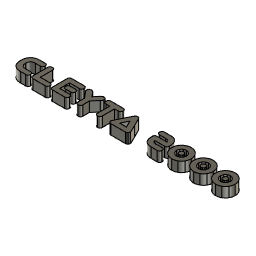
cleyta - letras v1 (Autodesk Fusion 360 design; units mm, degrees)
Autodesk Fusion 360 part; units mm, degrees
sketch "Sketch1" plane through (0, 0, 0) normal (0, 0, 1) x (1, 0, 0)
  spline S0 degree 3 poles (59.1791, -37.5966) (59.1791, -37.7184) (59.1478, -37.8357) (59.086, -37.9476) knots 0 0 0 0 1 1 1 1
  line L0 (68.0423, 3.3248) -> (69.0237, 3.3223)
  spline S1 degree 3 poles (69.0237, 3.3223) (69.3487, 3.3173) (69.5125, 3.1554) (69.5144, 2.8366) knots 0 0 0 0 1 1 1 1
  spline S2 degree 3 poles (69.5144, 2.8366) (69.5125, 2.5059) (69.3481, 2.3415) (69.0212, 2.3434) knots 0 0 0 0 1 1 1 1
  line L1 (69.0212, 2.3434) -> (68.0448, 2.3409)
  spline S3 degree 3 poles (68.0448, 2.3409) (67.3921, 2.3459) (67.0658, 2.0202) (67.0658, 1.3644) knots 0 0 0 0 1 1 1 1
  spline S4 degree 3 poles (67.0658, 1.3644) (67.0658, 0.7131) (67.3921, 0.3862) (68.0448, 0.383) knots 0 0 0 0 1 1 1 1
  line L2 (68.0448, 0.383) -> (69.0212, 0.383)
  spline S5 degree 3 poles (69.0212, 0.383) (69.3481, 0.3762) (69.5119, 0.2143) (69.5119, -0.1027) knots 0 0 0 0 1 1 1 1
  spline S6 degree 3 poles (69.5119, -0.1027) (69.5119, -0.4302) (69.35, -0.5946) (69.0262, -0.5959) knots 0 0 0 0 1 1 1 1
  line L3 (69.0262, -0.5959) -> (68.0448, -0.5959)
  spline S7 degree 3 poles (68.0448, -0.5959) (66.7377, -0.5959) (66.0832, 0.058) (66.0819, 1.3669) knots 0 0 0 0 1 1 1 1
  spline S8 degree 3 poles (66.0819, 1.3669) (66.0819, 2.6734) (66.7352, 3.326) (68.0423, 3.3248) knots 0 0 0 0 1 1 1 1
  spline S9 degree 3 poles (70.4933, 3.3298) (70.8221, 3.321) (70.9878, 3.161) (70.9915, 2.849) knots 0 0 0 0 1 1 1 1
  line L4 (70.9915, 2.849) -> (70.9865, 0.388)
  line L5 (70.9865, 0.388) -> (72.9344, 0.388)
  spline S10 degree 3 poles (72.9344, 0.388) (73.2644, 0.3862) (73.4301, 0.2211) (73.4301, -0.1077) knots 0 0 0 0 1 1 1 1
  spline S11 degree 3 poles (73.4301, -0.1077) (73.4282, -0.4302) (73.2663, -0.5928) (72.9444, -0.5959) knots 0 0 0 0 1 1 1 1
  line L6 (72.9444, -0.5959) -> (70.4933, -0.5959)
  spline S12 degree 3 poles (70.4933, -0.5959) (70.1676, -0.5959) (70.0039, -0.4377) (70.0026, -0.1201) knots 0 0 0 0 1 1 1 1
  line L7 (70.0026, -0.1201) -> (70.0026, 2.8341)
  spline S13 degree 3 poles (70.0026, 2.8341) (70.0039, 3.1579) (70.1676, 3.3229) (70.4933, 3.3298) knots 0 0 0 0 1 1 1 1
  line L8 (74.414, 3.3298) -> (76.8949, 3.3248)
  spline S14 degree 3 poles (76.8949, 3.3248) (77.2001, 3.3198) (77.3539, 3.161) (77.3557, 2.849) knots 0 0 0 0 1 1 1 1
  spline S15 degree 3 poles (77.3557, 2.849) (77.3557, 2.5152) (77.1901, 2.3459) (76.8601, 2.3409) knots 0 0 0 0 1 1 1 1
  line L9 (76.8601, 2.3409) -> (74.9072, 2.3409)
  line L10 (74.9072, 2.3409) -> (74.9072, 0.388)
  line L11 (74.9072, 0.388) -> (76.8551, 0.388)
  spline S16 degree 3 poles (76.8551, 0.388) (77.1851, 0.3862) (77.3508, 0.2211) (77.3508, -0.1077) knots 0 0 0 0 1 1 1 1
  spline S17 degree 3 poles (77.3508, -0.1077) (77.3489, -0.4302) (77.187, -0.5928) (76.865, -0.5959) knots 0 0 0 0 1 1 1 1
  line L12 (76.865, -0.5959) -> (74.414, -0.5959)
  spline S18 degree 3 poles (74.414, -0.5959) (74.0883, -0.5959) (73.9246, -0.4377) (73.9233, -0.1201) knots 0 0 0 0 1 1 1 1
  line L13 (73.9233, -0.1201) -> (73.9233, 2.8341)
  spline S19 degree 3 poles (73.9233, 2.8341) (73.9246, 3.1579) (74.0883, 3.3229) (74.414, 3.3298) knots 0 0 0 0 1 1 1 1
  spline S20 degree 3 poles (75.1414, 1.3545) (75.1445, 1.6795) (75.3064, 1.8452) (75.6271, 1.8502) knots 0 0 0 0 1 1 1 1
  line L14 (75.6271, 1.8502) -> (76.6135, 1.8502)
  spline S21 degree 3 poles (76.6135, 1.8502) (76.9404, 1.8464) (77.1067, 1.6833) (77.1116, 1.3595) knots 0 0 0 0 1 1 1 1
  spline S22 degree 3 poles (77.1116, 1.3595) (77.1048, 1.0319) (76.9398, 0.8688) (76.616, 0.8688) knots 0 0 0 0 1 1 1 1
  line L15 (76.616, 0.8688) -> (75.6296, 0.8688)
  spline S23 degree 3 poles (75.6296, 0.8688) (75.3058, 0.8669) (75.1426, 1.0288) (75.1414, 1.3545) knots 0 0 0 0 1 1 1 1
  spline S24 degree 3 poles (78.3422, 3.3347) (78.5047, 3.3347) (78.6274, 3.2936) (78.7108, 3.2127) knots 0 0 0 0 1 1 1 1
  spline S25 degree 3 poles (78.7108, 3.2127) (78.7936, 3.133) (79.0845, 2.7917) (79.5826, 2.1889) knots 0 0 0 0 1 1 1 1
  spline S26 degree 3 poles (79.5826, 2.1889) (80.0889, 2.8017) (80.3834, 3.1479) (80.4669, 3.2276) knots 0 0 0 0 1 1 1 1
  spline S27 degree 3 poles (80.4669, 3.2276) (80.5497, 3.3073) (80.6724, 3.3472) (80.8355, 3.3472) knots 0 0 0 0 1 1 1 1
  spline S28 degree 3 poles (80.8355, 3.3472) (80.995, 3.3472) (81.1176, 3.3055) (81.2042, 3.2226) knots 0 0 0 0 1 1 1 1
  spline S29 degree 3 poles (81.2042, 3.2226) (81.2901, 3.1392) (81.3312, 3.0159) (81.3262, 2.8515) knots 0 0 0 0 1 1 1 1
  spline S30 degree 3 poles (81.3262, 2.8515) (81.3262, 2.6784) (81.2397, 2.5165) (81.0672, 2.3658) knots 0 0 0 0 1 1 1 1
  line L16 (81.0672, 2.3658) -> (80.0634, 1.1951)
  line L17 (80.0634, 1.1951) -> (80.0609, -0.1077)
  spline S31 degree 3 poles (80.0609, -0.1077) (80.054, -0.4284) (79.8896, -0.5909) (79.5677, -0.5959) knots 0 0 0 0 1 1 1 1
  spline S32 degree 3 poles (79.5677, -0.5959) (79.2439, -0.604) (79.082, -0.4365) (79.082, -0.0927) knots 0 0 0 0 1 1 1 1
  line L18 (79.082, -0.0927) -> (79.077, 1.2001)
  line L19 (79.077, 1.2001) -> (78.1105, 2.3508)
  spline S33 degree 3 poles (78.1105, 2.3508) (77.9374, 2.5034) (77.8515, 2.6659) (77.8515, 2.8391) knots 0 0 0 0 1 1 1 1
  spline S34 degree 3 poles (77.8515, 2.8391) (77.8465, 3.0047) (77.8863, 3.1286) (77.971, 3.2102) knots 0 0 0 0 1 1 1 1
  spline S35 degree 3 poles (77.971, 3.2102) (78.057, 3.293) (78.1809, 3.3347) (78.3422, 3.3347) knots 0 0 0 0 1 1 1 1
  line L20 (82.2603, 3.3298) -> (84.7412, 3.3248)
  spline S36 degree 3 poles (84.7412, 3.3248) (85.0463, 3.3198) (85.2001, 3.161) (85.202, 2.849) knots 0 0 0 0 1 1 1 1
  spline S37 degree 3 poles (85.202, 2.849) (85.202, 2.5152) (85.0364, 2.3459) (84.7063, 2.3409) knots 0 0 0 0 1 1 1 1
  line L21 (84.7063, 2.3409) -> (83.974, 2.3409)
  line L22 (83.974, 2.3409) -> (83.9765, -0.1077)
  spline S38 degree 3 poles (83.9765, -0.1077) (83.9728, -0.4302) (83.8084, -0.5928) (83.4833, -0.5959) knots 0 0 0 0 1 1 1 1
  spline S39 degree 3 poles (83.4833, -0.5959) (83.1558, -0.5959) (82.9926, -0.4377) (82.9926, -0.1201) knots 0 0 0 0 1 1 1 1
  line L23 (82.9926, -0.1201) -> (82.9951, 2.3409)
  line L24 (82.9951, 2.3409) -> (82.2603, 2.3409)
  spline S40 degree 3 poles (82.2603, 2.3409) (81.9327, 2.3409) (81.7696, 2.5053) (81.7696, 2.8341) knots 0 0 0 0 1 1 1 1
  spline S41 degree 3 poles (81.7696, 2.8341) (81.7708, 3.1579) (81.9346, 3.3229) (82.2603, 3.3298) knots 0 0 0 0 1 1 1 1
  spline S42 degree 3 poles (86.1835, -0.5984) (86.1, -0.5984) (86.0197, -0.5778) (85.9418, -0.5361) knots 0 0 0 0 1 1 1 1
  spline S43 degree 3 poles (85.9418, -0.5361) (85.8634, -0.495) (85.8024, -0.4352) (85.7575, -0.3567) knots 0 0 0 0 1 1 1 1
  spline S44 degree 3 poles (85.7575, -0.3567) (85.7139, -0.277) (85.6928, -0.1942) (85.6928, -0.1077) knots 0 0 0 0 1 1 1 1
  spline S45 degree 3 poles (85.6928, -0.1077) (85.6928, -0.023) (85.9369, 0.5101) (86.4251, 1.4915) knots 0 0 0 0 1 1 1 1
  spline S46 degree 3 poles (86.4251, 1.4915) (86.9145, 2.4741) (87.1804, 3.0047) (87.2222, 3.0832) knots 0 0 0 0 1 1 1 1
  spline S47 degree 3 poles (87.2222, 3.0832) (87.2651, 3.161) (87.3255, 3.2214) (87.404, 3.265) knots 0 0 0 0 1 1 1 1
  spline S48 degree 3 poles (87.404, 3.265) (87.4818, 3.308) (87.564, 3.3298) (87.6506, 3.3298) knots 0 0 0 0 1 1 1 1
  spline S49 degree 3 poles (87.6506, 3.3298) (87.7353, 3.3298) (87.8156, 3.308) (87.8922, 3.265) knots 0 0 0 0 1 1 1 1
  spline S50 degree 3 poles (87.8922, 3.265) (87.97, 3.2214) (88.0304, 3.161) (88.074, 3.0832) knots 0 0 0 0 1 1 1 1
  spline S51 degree 3 poles (88.074, 3.0832) (88.117, 3.0047) (88.3842, 2.4741) (88.8761, 1.4915) knots 0 0 0 0 1 1 1 1
  spline S52 degree 3 poles (88.8761, 1.4915) (89.3674, 0.5101) (89.6134, -0.023) (89.6134, -0.1077) knots 0 0 0 0 1 1 1 1
  spline S53 degree 3 poles (89.6134, -0.1077) (89.6134, -0.1942) (89.591, -0.277) (89.5461, -0.3567) knots 0 0 0 0 1 1 1 1
  spline S54 degree 3 poles (89.5461, -0.3567) (89.5026, -0.4352) (89.4415, -0.495) (89.3618, -0.5361) knots 0 0 0 0 1 1 1 1
  spline S55 degree 3 poles (89.3618, -0.5361) (89.2834, -0.5778) (89.2037, -0.5984) (89.1227, -0.5984) knots 0 0 0 0 1 1 1 1
  line L25 (89.1227, -0.5984) -> (86.1835, -0.5984)
  line L26 (88.3206, 0.3905) -> (87.6506, 1.7705)
  line L27 (87.6506, 1.7705) -> (86.9756, 0.3905)
  line L28 (86.9756, 0.3905) -> (88.3206, 0.3905)
  spline S56 degree 3 poles (94.2696, 3.3248) (95.4135, 3.326) (95.9864, 2.6728) (95.9883, 1.3644) knots 0 0 0 0 1 1 1 1
  spline S57 degree 3 poles (95.9883, 1.3644) (95.9895, 1.0369) (95.8264, 0.8744) (95.4976, 0.8762) knots 0 0 0 0 1 1 1 1
  line L29 (95.4976, 0.8762) -> (93.5347, 0.8787)
  spline S58 degree 3 poles (93.5347, 0.8787) (93.5379, 0.5499) (93.782, 0.3843) (94.2671, 0.383) knots 0 0 0 0 1 1 1 1
  line L30 (94.2671, 0.383) -> (95.5001, 0.388)
  spline S59 degree 3 poles (95.5001, 0.388) (95.8201, 0.3862) (95.9833, 0.2218) (95.9883, -0.1052) knots 0 0 0 0 1 1 1 1
  spline S60 degree 3 poles (95.9883, -0.1052) (95.9864, -0.434) (95.8226, -0.5971) (95.4976, -0.5959) knots 0 0 0 0 1 1 1 1
  line L31 (95.4976, -0.5959) -> (94.2745, -0.5959)
  spline S61 degree 3 poles (94.2745, -0.5959) (93.1269, -0.5946) (92.5521, 0.0599) (92.5508, 1.3669) knots 0 0 0 0 1 1 1 1
  spline S62 degree 3 poles (92.5508, 1.3669) (92.5521, 1.6908) (92.7159, 1.8533) (93.0416, 1.8552) knots 0 0 0 0 1 1 1 1
  line L32 (93.0416, 1.8552) -> (95.0044, 1.8527)
  spline S63 degree 3 poles (95.0044, 1.8527) (95.0044, 2.1796) (94.7628, 2.3421) (94.2795, 2.3409) knots 0 0 0 0 1 1 1 1
  line L33 (94.2795, 2.3409) -> (93.0465, 2.3409)
  spline S64 degree 3 poles (93.0465, 2.3409) (92.7227, 2.349) (92.5571, 2.514) (92.5508, 2.8366) knots 0 0 0 0 1 1 1 1
  spline S65 degree 3 poles (92.5508, 2.8366) (92.5589, 3.1635) (92.724, 3.326) (93.0465, 3.3248) knots 0 0 0 0 1 1 1 1
  line L34 (93.0465, 3.3248) -> (94.2696, 3.3248)
  spline S66 degree 3 poles (98.4343, 3.3248) (98.7631, 3.3248) (99.0832, 3.2401) (99.3958, 3.0707) knots 0 0 0 0 1 1 1 1
  spline S67 degree 3 poles (99.3958, 3.0707) (99.7096, 2.9013) (99.955, 2.6585) (100.1331, 2.3434) knots 0 0 0 0 1 1 1 1
  spline S68 degree 3 poles (100.1331, 2.3434) (100.3106, 2.0295) (100.3996, 1.702) (100.3996, 1.362) knots 0 0 0 0 1 1 1 1
  spline S69 degree 3 poles (100.3996, 1.362) (100.3996, 1.0213) (100.3131, 0.695) (100.1406, 0.383) knots 0 0 0 0 1 1 1 1
  spline S70 degree 3 poles (100.1406, 0.383) (99.9674, 0.0723) (99.7252, -0.1693) (99.4132, -0.3418) knots 0 0 0 0 1 1 1 1
  spline S71 degree 3 poles (99.4132, -0.3418) (99.1006, -0.5149) (98.7743, -0.6009) (98.4343, -0.6009) knots 0 0 0 0 1 1 1 1
  spline S72 degree 3 poles (98.4343, -0.6009) (98.0955, -0.6009) (97.7699, -0.5149) (97.4579, -0.3418) knots 0 0 0 0 1 1 1 1
  spline S73 degree 3 poles (97.4579, -0.3418) (97.1453, -0.1693) (96.903, 0.0723) (96.7305, 0.383) knots 0 0 0 0 1 1 1 1
  spline S74 degree 3 poles (96.7305, 0.383) (96.5574, 0.695) (96.4715, 1.0213) (96.4715, 1.362) knots 0 0 0 0 1 1 1 1
  spline S75 degree 3 poles (96.4715, 1.362) (96.4715, 1.702) (96.5587, 2.0295) (96.733, 2.3434) knots 0 0 0 0 1 1 1 1
  spline S76 degree 3 poles (96.733, 2.3434) (96.9086, 2.6585) (97.1527, 2.9013) (97.4654, 3.0707) knots 0 0 0 0 1 1 1 1
  spline S77 degree 3 poles (97.4654, 3.0707) (97.7792, 3.2401) (98.1018, 3.3248) (98.4343, 3.3248) knots 0 0 0 0 1 1 1 1
  spline S78 degree 3 poles (98.4368, 2.3483) (98.2705, 2.3483) (98.1092, 2.306) (97.9536, 2.2213) knots 0 0 0 0 1 1 1 1
  spline S79 degree 3 poles (97.9536, 2.2213) (97.7973, 2.1379) (97.6752, 2.0177) (97.5874, 1.8601) knots 0 0 0 0 1 1 1 1
  spline S80 degree 3 poles (97.5874, 1.8601) (97.499, 1.702) (97.4554, 1.5376) (97.4554, 1.3669) knots 0 0 0 0 1 1 1 1
  spline S81 degree 3 poles (97.4554, 1.3669) (97.4554, 1.1957) (97.4984, 1.0319) (97.5849, 0.8762) knots 0 0 0 0 1 1 1 1
  spline S82 degree 3 poles (97.5849, 0.8762) (97.6709, 0.7218) (97.7923, 0.601) (97.9486, 0.5151) knots 0 0 0 0 1 1 1 1
  spline S83 degree 3 poles (97.9486, 0.5151) (98.1043, 0.4285) (98.2674, 0.3855) (98.4368, 0.3855) knots 0 0 0 0 1 1 1 1
  spline S84 degree 3 poles (98.4368, 0.3855) (98.6074, 0.3855) (98.7712, 0.4285) (98.9275, 0.5151) knots 0 0 0 0 1 1 1 1
  spline S85 degree 3 poles (98.9275, 0.5151) (99.0832, 0.601) (99.2046, 0.7218) (99.2912, 0.8762) knots 0 0 0 0 1 1 1 1
  spline S86 degree 3 poles (99.2912, 0.8762) (99.3771, 1.0319) (99.4207, 1.1957) (99.4207, 1.3669) knots 0 0 0 0 1 1 1 1
  spline S87 degree 3 poles (99.4207, 1.3669) (99.4207, 1.5376) (99.3765, 1.702) (99.2887, 1.8601) knots 0 0 0 0 1 1 1 1
  spline S88 degree 3 poles (99.2887, 1.8601) (99.2003, 2.0177) (99.0776, 2.1379) (98.92, 2.2213) knots 0 0 0 0 1 1 1 1
  spline S89 degree 3 poles (98.92, 2.2213) (98.7637, 2.306) (98.6024, 2.3483) (98.4368, 2.3483) knots 0 0 0 0 1 1 1 1
  spline S90 degree 3 poles (98.4343, 1.8452) (98.5153, 1.8452) (98.5943, 1.8234) (98.6709, 1.7804) knots 0 0 0 0 1 1 1 1
  spline S91 degree 3 poles (98.6709, 1.7804) (98.7488, 1.7387) (98.8092, 1.6789) (98.8528, 1.6011) knots 0 0 0 0 1 1 1 1
  spline S92 degree 3 poles (98.8528, 1.6011) (98.8976, 1.5245) (98.92, 1.4429) (98.92, 1.357) knots 0 0 0 0 1 1 1 1
  spline S93 degree 3 poles (98.92, 1.357) (98.92, 1.2723) (98.8982, 1.1907) (98.8553, 1.1129) knots 0 0 0 0 1 1 1 1
  spline S94 degree 3 poles (98.8553, 1.1129) (98.8117, 1.0363) (98.7519, 0.9765) (98.6759, 0.9335) knots 0 0 0 0 1 1 1 1
  spline S95 degree 3 poles (98.6759, 0.9335) (98.5993, 0.8918) (98.519, 0.8713) (98.4343, 0.8713) knots 0 0 0 0 1 1 1 1
  spline S96 degree 3 poles (98.4343, 0.8713) (98.3477, 0.8713) (98.2655, 0.8918) (98.1877, 0.9335) knots 0 0 0 0 1 1 1 1
  spline S97 degree 3 poles (98.1877, 0.9335) (98.1111, 0.9765) (98.0513, 1.0363) (98.0084, 1.1129) knots 0 0 0 0 1 1 1 1
  spline S98 degree 3 poles (98.0084, 1.1129) (97.9666, 1.1907) (97.9461, 1.2723) (97.9461, 1.357) knots 0 0 0 0 1 1 1 1
  spline S99 degree 3 poles (97.9461, 1.357) (97.9461, 1.4429) (97.9673, 1.5245) (98.0109, 1.6011) knots 0 0 0 0 1 1 1 1
  spline S100 degree 3 poles (98.0109, 1.6011) (98.0538, 1.6789) (98.1136, 1.7387) (98.1902, 1.7804) knots 0 0 0 0 1 1 1 1
  spline S101 degree 3 poles (98.1902, 1.7804) (98.268, 1.8234) (98.3496, 1.8452) (98.4343, 1.8452) knots 0 0 0 0 1 1 1 1
  spline S102 degree 3 poles (102.8503, 3.3248) (103.1791, 3.3248) (103.4992, 3.2401) (103.8118, 3.0707) knots 0 0 0 0 1 1 1 1
  spline S103 degree 3 poles (103.8118, 3.0707) (104.1256, 2.9013) (104.371, 2.6585) (104.5491, 2.3434) knots 0 0 0 0 1 1 1 1
  spline S104 degree 3 poles (104.5491, 2.3434) (104.7265, 2.0295) (104.8156, 1.702) (104.8156, 1.362) knots 0 0 0 0 1 1 1 1
  spline S105 degree 3 poles (104.8156, 1.362) (104.8156, 1.0213) (104.729, 0.695) (104.5565, 0.383) knots 0 0 0 0 1 1 1 1
  spline S106 degree 3 poles (104.5565, 0.383) (104.3834, 0.0723) (104.1412, -0.1693) (103.8292, -0.3418) knots 0 0 0 0 1 1 1 1
  spline S107 degree 3 poles (103.8292, -0.3418) (103.5166, -0.5149) (103.1903, -0.6009) (102.8503, -0.6009) knots 0 0 0 0 1 1 1 1
  spline S108 degree 3 poles (102.8503, -0.6009) (102.5115, -0.6009) (102.1858, -0.5149) (101.8739, -0.3418) knots 0 0 0 0 1 1 1 1
  spline S109 degree 3 poles (101.8739, -0.3418) (101.5613, -0.1693) (101.319, 0.0723) (101.1465, 0.383) knots 0 0 0 0 1 1 1 1
  spline S110 degree 3 poles (101.1465, 0.383) (100.9734, 0.695) (100.8875, 1.0213) (100.8875, 1.362) knots 0 0 0 0 1 1 1 1
  spline S111 degree 3 poles (100.8875, 1.362) (100.8875, 1.702) (100.9747, 2.0295) (101.149, 2.3434) knots 0 0 0 0 1 1 1 1
  spline S112 degree 3 poles (101.149, 2.3434) (101.3246, 2.6585) (101.5687, 2.9013) (101.8813, 3.0707) knots 0 0 0 0 1 1 1 1
  spline S113 degree 3 poles (101.8813, 3.0707) (102.1952, 3.2401) (102.5178, 3.3248) (102.8503, 3.3248) knots 0 0 0 0 1 1 1 1
  spline S114 degree 3 poles (102.8528, 2.3483) (102.6865, 2.3483) (102.5252, 2.306) (102.3695, 2.2213) knots 0 0 0 0 1 1 1 1
  spline S115 degree 3 poles (102.3695, 2.2213) (102.2132, 2.1379) (102.0912, 2.0177) (102.0034, 1.8601) knots 0 0 0 0 1 1 1 1
  spline S116 degree 3 poles (102.0034, 1.8601) (101.915, 1.702) (101.8714, 1.5376) (101.8714, 1.3669) knots 0 0 0 0 1 1 1 1
  spline S117 degree 3 poles (101.8714, 1.3669) (101.8714, 1.1957) (101.9143, 1.0319) (102.0009, 0.8762) knots 0 0 0 0 1 1 1 1
  spline S118 degree 3 poles (102.0009, 0.8762) (102.0868, 0.7218) (102.2083, 0.601) (102.3646, 0.5151) knots 0 0 0 0 1 1 1 1
  spline S119 degree 3 poles (102.3646, 0.5151) (102.5202, 0.4285) (102.6834, 0.3855) (102.8528, 0.3855) knots 0 0 0 0 1 1 1 1
  spline S120 degree 3 poles (102.8528, 0.3855) (103.0234, 0.3855) (103.1872, 0.4285) (103.3435, 0.5151) knots 0 0 0 0 1 1 1 1
  spline S121 degree 3 poles (103.3435, 0.5151) (103.4992, 0.601) (103.6206, 0.7218) (103.7071, 0.8762) knots 0 0 0 0 1 1 1 1
  spline S122 degree 3 poles (103.7071, 0.8762) (103.7931, 1.0319) (103.8367, 1.1957) (103.8367, 1.3669) knots 0 0 0 0 1 1 1 1
  spline S123 degree 3 poles (103.8367, 1.3669) (103.8367, 1.5376) (103.7925, 1.702) (103.7047, 1.8601) knots 0 0 0 0 1 1 1 1
  spline S124 degree 3 poles (103.7047, 1.8601) (103.6162, 2.0177) (103.4936, 2.1379) (103.336, 2.2213) knots 0 0 0 0 1 1 1 1
  spline S125 degree 3 poles (103.336, 2.2213) (103.1797, 2.306) (103.0184, 2.3483) (102.8528, 2.3483) knots 0 0 0 0 1 1 1 1
  spline S126 degree 3 poles (102.8503, 1.8452) (102.9312, 1.8452) (103.0103, 1.8234) (103.0869, 1.7804) knots 0 0 0 0 1 1 1 1
  spline S127 degree 3 poles (103.0869, 1.7804) (103.1648, 1.7387) (103.2252, 1.6789) (103.2688, 1.6011) knots 0 0 0 0 1 1 1 1
  spline S128 degree 3 poles (103.2688, 1.6011) (103.3136, 1.5245) (103.336, 1.4429) (103.336, 1.357) knots 0 0 0 0 1 1 1 1
  spline S129 degree 3 poles (103.336, 1.357) (103.336, 1.2723) (103.3142, 1.1907) (103.2712, 1.1129) knots 0 0 0 0 1 1 1 1
  spline S130 degree 3 poles (103.2712, 1.1129) (103.2277, 1.0363) (103.1679, 0.9765) (103.0919, 0.9335) knots 0 0 0 0 1 1 1 1
  spline S131 degree 3 poles (103.0919, 0.9335) (103.0153, 0.8918) (102.935, 0.8713) (102.8503, 0.8713) knots 0 0 0 0 1 1 1 1
  spline S132 degree 3 poles (102.8503, 0.8713) (102.7637, 0.8713) (102.6815, 0.8918) (102.6037, 0.9335) knots 0 0 0 0 1 1 1 1
  spline S133 degree 3 poles (102.6037, 0.9335) (102.5271, 0.9765) (102.4673, 1.0363) (102.4243, 1.1129) knots 0 0 0 0 1 1 1 1
  spline S134 degree 3 poles (102.4243, 1.1129) (102.3826, 1.1907) (102.3621, 1.2723) (102.3621, 1.357) knots 0 0 0 0 1 1 1 1
  spline S135 degree 3 poles (102.3621, 1.357) (102.3621, 1.4429) (102.3832, 1.5245) (102.4268, 1.6011) knots 0 0 0 0 1 1 1 1
  spline S136 degree 3 poles (102.4268, 1.6011) (102.4698, 1.6789) (102.5296, 1.7387) (102.6062, 1.7804) knots 0 0 0 0 1 1 1 1
  spline S137 degree 3 poles (102.6062, 1.7804) (102.684, 1.8234) (102.7656, 1.8452) (102.8503, 1.8452) knots 0 0 0 0 1 1 1 1
  spline S138 degree 3 poles (107.2663, 3.3248) (107.5951, 3.3248) (107.9151, 3.2401) (108.2277, 3.0707) knots 0 0 0 0 1 1 1 1
  spline S139 degree 3 poles (108.2277, 3.0707) (108.5416, 2.9013) (108.7869, 2.6585) (108.965, 2.3434) knots 0 0 0 0 1 1 1 1
  spline S140 degree 3 poles (108.965, 2.3434) (109.1425, 2.0295) (109.2316, 1.702) (109.2316, 1.362) knots 0 0 0 0 1 1 1 1
  spline S141 degree 3 poles (109.2316, 1.362) (109.2316, 1.0213) (109.145, 0.695) (108.9725, 0.383) knots 0 0 0 0 1 1 1 1
  spline S142 degree 3 poles (108.9725, 0.383) (108.7994, 0.0723) (108.5572, -0.1693) (108.2452, -0.3418) knots 0 0 0 0 1 1 1 1
  spline S143 degree 3 poles (108.2452, -0.3418) (107.9326, -0.5149) (107.6063, -0.6009) (107.2663, -0.6009) knots 0 0 0 0 1 1 1 1
  spline S144 degree 3 poles (107.2663, -0.6009) (106.9275, -0.6009) (106.6018, -0.5149) (106.2898, -0.3418) knots 0 0 0 0 1 1 1 1
  spline S145 degree 3 poles (106.2898, -0.3418) (105.9772, -0.1693) (105.735, 0.0723) (105.5625, 0.383) knots 0 0 0 0 1 1 1 1
  spline S146 degree 3 poles (105.5625, 0.383) (105.3894, 0.695) (105.3035, 1.0213) (105.3035, 1.362) knots 0 0 0 0 1 1 1 1
  spline S147 degree 3 poles (105.3035, 1.362) (105.3035, 1.702) (105.3906, 2.0295) (105.565, 2.3434) knots 0 0 0 0 1 1 1 1
  spline S148 degree 3 poles (105.565, 2.3434) (105.7406, 2.6585) (105.9847, 2.9013) (106.2973, 3.0707) knots 0 0 0 0 1 1 1 1
  spline S149 degree 3 poles (106.2973, 3.0707) (106.6112, 3.2401) (106.9337, 3.3248) (107.2663, 3.3248) knots 0 0 0 0 1 1 1 1
  spline S150 degree 3 poles (107.2688, 2.3483) (107.1025, 2.3483) (106.9412, 2.306) (106.7855, 2.2213) knots 0 0 0 0 1 1 1 1
  spline S151 degree 3 poles (106.7855, 2.2213) (106.6292, 2.1379) (106.5072, 2.0177) (106.4194, 1.8601) knots 0 0 0 0 1 1 1 1
  spline S152 degree 3 poles (106.4194, 1.8601) (106.3309, 1.702) (106.2873, 1.5376) (106.2873, 1.3669) knots 0 0 0 0 1 1 1 1
  spline S153 degree 3 poles (106.2873, 1.3669) (106.2873, 1.1957) (106.3303, 1.0319) (106.4169, 0.8762) knots 0 0 0 0 1 1 1 1
  spline S154 degree 3 poles (106.4169, 0.8762) (106.5028, 0.7218) (106.6242, 0.601) (106.7805, 0.5151) knots 0 0 0 0 1 1 1 1
  spline S155 degree 3 poles (106.7805, 0.5151) (106.9362, 0.4285) (107.0994, 0.3855) (107.2688, 0.3855) knots 0 0 0 0 1 1 1 1
  spline S156 degree 3 poles (107.2688, 0.3855) (107.4394, 0.3855) (107.6032, 0.4285) (107.7595, 0.5151) knots 0 0 0 0 1 1 1 1
  spline S157 degree 3 poles (107.7595, 0.5151) (107.9151, 0.601) (108.0366, 0.7218) (108.1231, 0.8762) knots 0 0 0 0 1 1 1 1
  spline S158 degree 3 poles (108.1231, 0.8762) (108.2091, 1.0319) (108.2527, 1.1957) (108.2527, 1.3669) knots 0 0 0 0 1 1 1 1
  spline S159 degree 3 poles (108.2527, 1.3669) (108.2527, 1.5376) (108.2084, 1.702) (108.1206, 1.8601) knots 0 0 0 0 1 1 1 1
  spline S160 degree 3 poles (108.1206, 1.8601) (108.0322, 2.0177) (107.9095, 2.1379) (107.752, 2.2213) knots 0 0 0 0 1 1 1 1
  spline S161 degree 3 poles (107.752, 2.2213) (107.5957, 2.306) (107.4344, 2.3483) (107.2688, 2.3483) knots 0 0 0 0 1 1 1 1
  spline S162 degree 3 poles (107.2663, 1.8452) (107.3472, 1.8452) (107.4263, 1.8234) (107.5029, 1.7804) knots 0 0 0 0 1 1 1 1
  spline S163 degree 3 poles (107.5029, 1.7804) (107.5807, 1.7387) (107.6411, 1.6789) (107.6847, 1.6011) knots 0 0 0 0 1 1 1 1
  spline S164 degree 3 poles (107.6847, 1.6011) (107.7296, 1.5245) (107.752, 1.4429) (107.752, 1.357) knots 0 0 0 0 1 1 1 1
  spline S165 degree 3 poles (107.752, 1.357) (107.752, 1.2723) (107.7302, 1.1907) (107.6872, 1.1129) knots 0 0 0 0 1 1 1 1
  spline S166 degree 3 poles (107.6872, 1.1129) (107.6436, 1.0363) (107.5839, 0.9765) (107.5079, 0.9335) knots 0 0 0 0 1 1 1 1
  spline S167 degree 3 poles (107.5079, 0.9335) (107.4313, 0.8918) (107.351, 0.8713) (107.2663, 0.8713) knots 0 0 0 0 1 1 1 1
  spline S168 degree 3 poles (107.2663, 0.8713) (107.1797, 0.8713) (107.0975, 0.8918) (107.0197, 0.9335) knots 0 0 0 0 1 1 1 1
  spline S169 degree 3 poles (107.0197, 0.9335) (106.9431, 0.9765) (106.8833, 1.0363) (106.8403, 1.1129) knots 0 0 0 0 1 1 1 1
  spline S170 degree 3 poles (106.8403, 1.1129) (106.7986, 1.1907) (106.7781, 1.2723) (106.7781, 1.357) knots 0 0 0 0 1 1 1 1
  spline S171 degree 3 poles (106.7781, 1.357) (106.7781, 1.4429) (106.7992, 1.5245) (106.8428, 1.6011) knots 0 0 0 0 1 1 1 1
  spline S172 degree 3 poles (106.8428, 1.6011) (106.8858, 1.6789) (106.9456, 1.7387) (107.0222, 1.7804) knots 0 0 0 0 1 1 1 1
  spline S173 degree 3 poles (107.0222, 1.7804) (107.1, 1.8234) (107.1816, 1.8452) (107.2663, 1.8452) knots 0 0 0 0 1 1 1 1
extrude "Extrude1" add sketch "Sketch1" along normal blind 2 makes body 1 at (74.2513, 1.034, 0) makes body 2 at (87.8756, -0.2687, 0) makes body 3 at (99.9148, 2.0502, 0) makes body 4 at (102.7664, 1.3362, 0) makes body 5 at (104.3308, 2.0502, 0) makes body 6 at (83.6585, 2.9985, 0) makes body 7 at (70.3306, 1.034, 0) makes body 8 at (76.2872, 0.8688, 0.6667) makes body 9 at (93.8602, 1.5288, 0) makes body 10 at (98.3504, 1.3362, 0) makes body 11 at (107.1824, 1.3362, 0) makes body 12 at (108.7467, 2.0502, 0) makes body 13 at (80.2377, 1.9166, 0) makes body 14 at (68.6974, -0.2696, 0)
